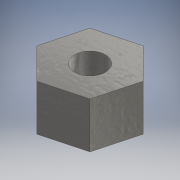
# Autodesk Inventor part: m2_nut
Saved by Autodesk Inventor 2017 (Build 210142000, 142)
## iProperties
Created: 2018-04-08
Part Number: m2_nut
Material: Steel, Galvanized
Document SubType Name: Modeling
Designer: Roland
Density: 7.85 g/cm^3
Appearance: Galvanized
Author: Roland
Autodesk Inventor part; units mm, degrees
ref_plane "YZ Plane" through (0, 0, 0) normal (1, 0, 0) x (0, 1, 0)
ref_plane "XZ Plane" through (0, 0, 0) normal (0, 1, 0) x (-1, 0, 0)
ref_plane "XY Plane" through (0, 0, 0) normal (0, 0, 1) x (1, 0, 0)
sketch "Sketch1" plane through (0, 0, 0) normal (0, 0, 1) x (1, 0, 0)
  line L0 (-2, 2) -> (0.7321, 2.7321)
  line L1 (0.7321, 2.7321) -> (2.7321, 0.7321)
  line L2 (2.7321, 0.7321) -> (2, -2)
  line L3 (2, -2) -> (-0.7321, -2.7321)
  line L4 (-0.7321, -2.7321) -> (-2.7321, -0.7321)
  line L5 (-2.7321, -0.7321) -> (-2, 2)
  circle A0 centre (0, 0) radius 1
  dimension "d2" = 2
  constraints: 12 end point, 3 coincident, 1 centre point, 13 other
  measures "d2" diameter of A0
extrude "Extrusion1" add sketch "Sketch1" along normal blind 3
body "Solid1"
